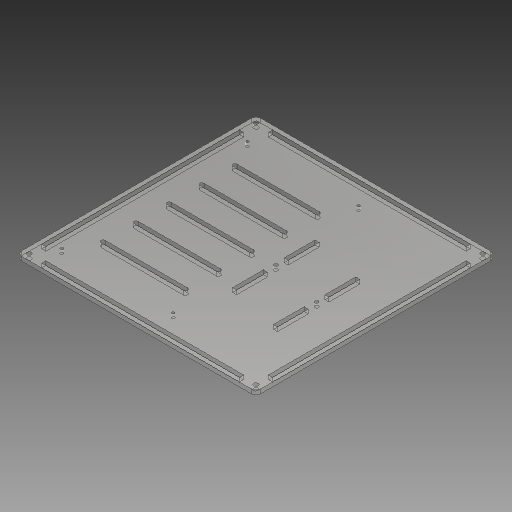
# Autodesk Inventor part: bottom
Saved by Autodesk Inventor 2019 (Build 230136000, 136)
## iProperties
Created: 2018-04-27
Part Number: bottom
Material: Polycarbonate, Clear
Document SubType Name: Modeling
Designer: Phil Erle
Density: 1.2 g/cm^3
Appearance: Polycarbonate - Clear
Author: Phil Erle
Autodesk Inventor part; units mm, degrees
ref_plane "YZ Plane" through (0, 0, 0) normal (1, 0, 0) x (0, 1, 0)
ref_plane "XZ Plane" through (0, 0, 0) normal (0, 1, 0) x (-1, 0, 0)
ref_plane "XY Plane" through (0, 0, 0) normal (0, 0, 1) x (1, 0, 0)
sketch "Sketch1" plane through (0, 0, 0) normal (0, 0, 1) x (1, 0, 0)
  line L0 (-145, -145) -> (145, -145)
  line L1 (145, -145) -> (145, 145)
  line L2 (145, 145) -> (-145, 145)
  line L3 (-145, 145) -> (-145, -145)
  line L4 (-145, -145) -> (145, 145) construction
  line L5 (145, -145) -> (-145, 145) construction
  point P0 (0, 0)
  dimension "d0" = 290
  dimension "d1" = 290
  constraints: 12 end point, 2 midpoint, 2 parallel, 1 horizontal, 1 perpendicular
  measures "d0" distance of L2.end L1.end
  measures "d1" distance of L1.end L0.end
extrude "Extrusion1" add sketch "Sketch1" along normal blind 5
sketch "Sketch2" plane through (0, 0, 5) normal (0, 0, 1) x (1, 0, 0)
  line L0 (-137.5, -137.5) -> (137.5, -137.5) construction
  line L1 (137.5, -137.5) -> (137.5, 137.5) construction
  line L2 (137.5, 137.5) -> (-137.5, 137.5) construction
  line L3 (-137.5, 137.5) -> (-137.5, -137.5) construction
  line L4 (-137.5, -137.5) -> (137.5, 137.5) construction
  line L5 (137.5, -137.5) -> (-137.5, 137.5) construction
  point P0 (0, 0)
  dimension "d4" = 275
  dimension "d5" = 275
  constraints: 12 end point, 4 coincident, 2 midpoint, 2 parallel, 1 horizontal, 1 perpendicular
  measures "d4" distance of L2.end L1.end
  measures "d5" distance of L1.end L0.end
hole "Hole1" at (-137.5, 137.5, 5) at (137.5, 137.5, 5) at (137.5, -137.5, 5) at (-137.5, -137.5, 5) direction (0, 0, -1) diameter 5.5 depth 8 tip angle 118 clearance for "Countersunk Flat Head Screw DIN EN ISO 2009" size "M5" standard "DIN"
sketch "Sketch3" plane through (0, 0, 5) normal (0, 0, 1) x (1, 0, 0)
  line L0 (-123, 112.5) -> (12, 112.5) construction
  line L1 (12, 112.5) -> (12, -112.5) construction
  line L2 (12, -112.5) -> (-123, -112.5) construction
  line L3 (-123, -112.5) -> (-123, 112.5) construction
  line L4 (-145, 145) -> (-145, -145) projected
  line L5 (145, -145) -> (145, 145) projected
  point P0 (0, 0)
  point P1 (12, 0)
  dimension "d13" = 135
  dimension "d34" = 225
  dimension "d35" = 22
  constraints: 8 end point, 4 coincident, 2 parallel, 1 horizontal, 1 horizontal alignment, 1 midpoint, 1 perpendicular
  measures "d13" distance of L0.start L0.end
  measures "d34" distance of L2.end L0.start
  measures "d35" distance between parallel lines of L4 L3
hole "Hole2" at (-123, 112.5, 5) at (12, 112.5, 5) at (12, -112.5, 5) at (-123, -112.5, 5) direction (0, 0, -1) diameter 3.4 depth 8 tip angle 118 clearance for "Countersunk Flat Head Screw DIN EN ISO 2009" size "M3" standard "DIN"
sketch "Sketch4" plane through (0, 0, 5) normal (0, 0, 1) x (1, 0, 0)
  line L0 (-140, 120) -> (-135, 120)
  line L1 (-135, 120) -> (-135, -120)
  line L2 (-135, -120) -> (-140, -120)
  line L3 (-140, -120) -> (-140, 120)
  line L4 (-120, -140) -> (120, -140)
  line L5 (120, -140) -> (120, -135)
  line L6 (120, -135) -> (-120, -135)
  line L7 (-120, -135) -> (-120, -140)
  line L8 (140, -120) -> (135, -120)
  line L9 (135, -120) -> (135, 120)
  line L10 (135, 120) -> (140, 120)
  line L11 (140, 120) -> (140, -120)
  line L12 (120, 140) -> (-120, 140)
  line L13 (-120, 140) -> (-120, 135)
  line L14 (-120, 135) -> (120, 135)
  line L15 (120, 135) -> (120, 140)
  line L16 (-145, 145) -> (-145, -145) projected
  line L17 (145, 145) -> (-145, 145) projected
  line L18 (145, -145) -> (145, 145) projected
  line L19 (-145, -145) -> (145, -145) projected
  point P0 (0, 0)
  point P1 (0, 135)
  point P2 (0, -135)
  point P3 (-135, 0)
  point P4 (135, 0)
  dimension "d21" = 240
  dimension "d22" = 240
  dimension "d23" = 5
  dimension "d24" = 5
  dimension "d25" = 5
  dimension "d26" = 5
  dimension "d27" = 5
  dimension "d28" = 5
  dimension "d29" = 5
  dimension "d30" = 5
  constraints: 32 end point, 8 parallel, 4 horizontal, 4 midpoint, 4 perpendicular, 3 point on line, 2 horizontal alignment, 2 vertical alignment
  measures "d21" distance of L12.start L12.end
  measures "d22" distance of L2.end L0.start
  measures "d23" distance of L0.start L0.end
  measures "d24" distance of L12.end L13.end
  measures "d25" distance of L9.end L10.end
  measures "d26" distance of L4.end L5.end
  measures "d27" distance between parallel lines of L16 L3
  measures "d28" distance between parallel lines of L17 L12
  measures "d29" distance between parallel lines of L18 L11
  measures "d30" distance between parallel lines of L19 L4
extrude "Extrusion2" cut sketch "Sketch4" against normal blind 10 contours L0 L1 L2 L3 | L7 L6 L5 L4 | L8 L9 L10 L11 | L15 L14 L13 L12
fillet "Fillet1" radius 6 4 edges at (-145, -145, 2.5) (145, -145, 2.5) (145, 145, 2.5) (-145, 145, 2.5)
sketch "Sketch6" plane through (0, 0, 5) normal (0, 0, 1) x (1, 0, 0)
  line L0 (135, -120) -> (135, 120) construction
  line L1 (21.5, 12.5) -> (26.5, 12.5)
  line L2 (26.5, 12.5) -> (26.5, 50)
  line L3 (26.5, 50) -> (21.5, 50)
  line L4 (21.5, 50) -> (21.5, 12.5)
  line L5 (21.5, -12.5) -> (26.5, -12.5)
  line L6 (26.5, -12.5) -> (26.5, -50)
  line L7 (26.5, -50) -> (21.5, -50)
  line L8 (21.5, -50) -> (21.5, -12.5)
  line L9 (90, -64) -> (85, -64)
  line L10 (85, -64) -> (85, -26.5)
  line L11 (85, -26.5) -> (90, -26.5)
  line L12 (90, -26.5) -> (90, -64)
  line L13 (90, -1.5) -> (85, -1.5)
  line L14 (85, -1.5) -> (85, 36)
  line L15 (85, 36) -> (90, 36)
  line L16 (90, 36) -> (90, -1.5)
  line L17 (21.5, -12.5) -> (21.5, 12.5) construction
  point P0 (0, 0)
  point P1 (21.5, 0)
  dimension "d95" = 5
  dimension "d96" = 37.5
  dimension "d97" = 37.5
  dimension "d98" = 5
  dimension "d99" = 25
  dimension "d100" = 21.5
  dimension "d101" = 37.5
  dimension "d102" = 5
  dimension "d103" = 37.5
  dimension "d104" = 25
  dimension "d105" = 58.5
  dimension "d113" = 14
  constraints: 34 end point, 8 parallel, 4 horizontal, 4 perpendicular, 2 point on line, 1 horizontal alignment, 1 midpoint, 1 vertical
  measures "d95" distance of L3.end L2.end
  measures "d96" distance of L3.end L1.start
  measures "d97" distance of L7.end L5.start
  measures "d98" distance of L6.end L7.end
  measures "d99" distance between parallel lines of L1 L5
  measures "d100" distance from line of point (0, 0) L8
  measures "d101" distance of L9.end L10.end
  measures "d102" distance of L9.start L9.end
  measures "d103" distance of L15.end L13.start
  measures "d104" distance between parallel lines of L13 L11
  measures "d105" distance between parallel lines of L6 L10
  measures "d113" distance between parallel lines of L9 L7
extrude "Extrusion3" cut sketch "Sketch6" against normal through all
sketch "Sketch7" plane through (0, 0, 5) normal (0, 0, 1) x (1, 0, 0)
  line L0 (21.5, 12.5) -> (21.5, 50) projected
  line L1 (26.5, 12.5) -> (21.5, 12.5) projected
  line L2 (85, -1.5) -> (85, 36) projected
  line L3 (90, -1.5) -> (85, -1.5) projected
  line L4 (85, -26.5) -> (90, -26.5) projected
  line L5 (21.5, -12.5) -> (26.5, -12.5) projected
  point P0 (0, 0)
  point P1 (24, 0)
  point P2 (87.5, -14)
  dimension "d107" = 2.5
  dimension "d108" = 2.5
  dimension "d109" = 25
  dimension "d110" = 12.5
  dimension "d111" = 25
  dimension "d112" = 12.5
  measures "d107" distance from line of L0 point (24, 0)
  measures "d108" distance from line of L2 point (87.5, -14)
  measures "d109" distance between parallel lines of L5 L1
  measures "d110" distance from line of L1 point (24, 0)
  measures "d111" distance between parallel lines of L4 L3
  measures "d112" distance from line of L3 point (87.5, -14)
hole "Hole3" at (24, 0, 5) at (87.5, -14, 5) direction (0, 0, -1) diameter 4.5 depth 8 tip angle 118 clearance for "Countersunk Flat Head Screw DIN EN ISO 2009" size "M4" standard "DIN"
sketch "Sketch11" plane through (0, 0, 5) normal (0, 0, 1) x (1, 0, 0)
  circle A0 centre (12, 112.5) radius 1.7 projected
  circle A1 centre (-123, 112.5) radius 1.7 projected
  circle A2 centre (-123, -112.5) radius 1.7 projected
  circle A3 centre (12, -112.5) radius 1.7 projected
  line L0 (12, 112.5) -> (-123, 112.5) construction
  line L1 (-123, 112.5) -> (-123, -112.5) construction
  line L2 (-123, -112.5) -> (12, -112.5) construction
  line L3 (12, -112.5) -> (12, 112.5) construction
  line L4 (-5.5, 0) -> (-105.5, 0) construction
  line L5 (-5.5, 2.5) -> (-105.5, 2.5)
  line L6 (-105.5, -2.5) -> (-5.5, -2.5)
  arc A4 (-5.5, -2.5) -> (-5.5, 2.5) centre (-5.5, 0) ccw
  arc A5 (-105.5, 2.5) -> (-105.5, -2.5) centre (-105.5, 0) ccw
  line L7 (-5.5, 40) -> (-105.5, 40) construction
  line L8 (-5.5, 42.5) -> (-105.5, 42.5)
  line L9 (-105.5, 37.5) -> (-5.5, 37.5)
  arc A6 (-5.5, 37.5) -> (-5.5, 42.5) centre (-5.5, 40) ccw
  arc A7 (-105.5, 42.5) -> (-105.5, 37.5) centre (-105.5, 40) ccw
  line L10 (-5.5, 80) -> (-105.5, 80) construction
  line L11 (-5.5, 82.5) -> (-105.5, 82.5)
  line L12 (-105.5, 77.5) -> (-5.5, 77.5)
  arc A8 (-5.5, 77.5) -> (-5.5, 82.5) centre (-5.5, 80) ccw
  arc A9 (-105.5, 82.5) -> (-105.5, 77.5) centre (-105.5, 80) ccw
  line L13 (-5.5, -37.5) -> (-105.5, -37.5)
  line L14 (-5.5, -40) -> (-105.5, -40) construction
  line L15 (-105.5, -42.5) -> (-5.5, -42.5)
  arc A10 (-5.5, -42.5) -> (-5.5, -37.5) centre (-5.5, -40) ccw
  arc A11 (-105.5, -37.5) -> (-105.5, -42.5) centre (-105.5, -40) ccw
  line L16 (-5.5, -77.5) -> (-105.5, -77.5)
  line L17 (-5.5, -80) -> (-105.5, -80) construction
  line L18 (-105.5, -82.5) -> (-5.5, -82.5)
  arc A12 (-5.5, -82.5) -> (-5.5, -77.5) centre (-5.5, -80) ccw
  arc A13 (-105.5, -77.5) -> (-105.5, -82.5) centre (-105.5, -80) ccw
  point P0 (0, 0)
  point P1 (-55.5, 0)
  point P2 (-55.5, 40)
  point P3 (-55.5, 80)
  point P4 (-55.5, -40)
  point P5 (-55.5, -80)
  dimension "d114" = 5
  dimension "d115" = 100
  dimension "d116" = 135
  dimension "d117" = 17.5
  dimension "d120" = 40
  dimension "d127" = 40
  constraints: 48 end point, 20 point on circle, 10 centre point, 4 tangent, 3 parallel, 2 horizontal, 2 vertical, 1 horizontal alignment, 1 midpoint, 1 perpendicular, 48 other
  measures "d114" distance between parallel lines of L6 L5
  measures "d115" distance of L6.start L6.end
  measures "d116" distance of L1.end L2.end
  measures "d117" distance from line of L3 L6.end
  measures "d120" distance of L5.start L8.start
  measures "d127" distance of L5.end L13.end
extrude "Extrusion4" cut sketch "Sketch11" against normal blind 10 contours A4 L6 A5 L5 | A6 L9 A7 L8 | A8 L12 A9 L11 | A10 L15 A11 L13 | A12 L18 A13 L16
equation "\"d110\" = 0.5 * d109"
equation "\"d112\" = 0.5 * d111"
equation "\"d117\" = -0.5 * d115 + 0.5 * d116"
body "Solid1"
